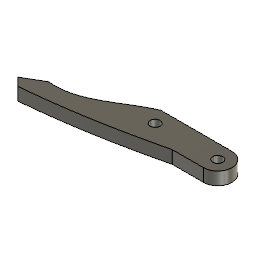
Gripper Holder 1.0 (Autodesk Fusion 360 design; units mm, degrees)
part number: 2026-08-19-22-23-44-975
Autodesk Fusion 360 part; units mm, degrees
sketch "Sketch1" plane through (0, 0, 0) normal (0, 0, 1) x (1, 0, 0)
  line L0 (-11, 0) -> (11, 0) construction
  circle A0 centre (-11, 0) radius 1.75
  circle A1 centre (-11, 0) radius 5
  circle A2 centre (11, 0) radius 1.75
  circle A3 centre (11, 0) radius 5
  line L1 (-11, 5) -> (11, 5)
  line L2 (11, -5) -> (-11, -5)
  dimension "d1" = 22
  dimension "d2" = 3.5
  dimension "d3" = 10
  dimension "d4" = 3.5
  dimension "d5" = 10
  constraint midpoint L0 origin
  constraint horizontal L0
  constraint coincident L0.start A0.centre
  constraint concentric A0 A1
  constraint coincident L0.end A2.centre
  constraint concentric A2 A3
  constraint coincident A1 L1.start
  constraint coincident A3 L1.end
  constraint tangent A3 L1
  constraint coincident A3 L2.start
  constraint coincident A1 L2.end
  constraint tangent A1 L2
  measures "d1" distance of L0.start L0.end
  measures "d2" diameter of A0
  measures "d3" diameter of A1
  measures "d4" diameter of A2
  measures "d5" diameter of A3
extrude "Extrude1" add sketch "Sketch1" along normal blind 4.5
sketch "Sketch2" plane through (0, 0, 4.5) normal (0, 0, 1) x (-1, 0, 0)
  circle A0 centre (-11, 0) radius 1.75
  circle A1 centre (11, 0) radius 1.75
  arc A2 (11, -5) -> (11, 5) centre (11, 0) ccw
  line L0 (11, 5) -> (-11, 5)
  arc A3 (-11, 5) -> (-11, -5) centre (-11, 0) ccw
  line L1 (-11, -5) -> (11, -5)
  line L2 (46.364, 12.87) -> (49.1808, 10.03)
  line L3 (49.1808, 10.03) -> (42.27, 6)
  line L4 (11, 0) -> (11, -5) construction
  spline S0 degree 5 poles (42.27, 6) (41.8597, 6.0483) (41.0377, 6.1242) (39.8004, 6.1754) (38.142, 6.1176) (36.0551, 5.832) (33.9568, 5.3324) (31.8528, 4.6259) (29.753, 3.7318) (27.6735, 2.6889) (25.6346, 1.5499) (23.6581, 0.3731) (21.7651, -0.7836) (19.9739, -1.8698) (18.2958, -2.85) (16.7347, -3.707) (15.5794, -4.2889) (14.7647, -4.667) (14.2444, -4.8933) (13.99, -5) knots 0 0 0 0 0 0 0.066667 0.133333 0.2 0.266667 0.333333 0.4 0.466667 0.533333 0.6 0.666667 0.733333 0.8 0.866667 0.933333 1 1 1 1 1 1
  line L5 (0, 0) -> (0, 5) construction
  spline S1 degree 5 poles (46.364, 12.87) (45.4848, 12.7904) (43.7223, 12.6243) (41.0656, 12.3544) (37.4975, 11.9526) (32.991, 11.3756) (28.4344, 10.7175) (23.8239, 9.9723) (19.158, 9.1377) (14.4396, 8.2182) (9.6729, 7.2207) (5.8243, 6.3656) (2.9193, 5.6943) (0.9744, 5.2336) (0, 5) knots 0 0 0 0 0 0 0.1 0.2 0.3 0.4 0.5 0.6 0.7 0.8 0.9 1 1 1 1 1 1
  line L6 (11, 0) -> (11, 5) construction
  line L7 (0, 5) -> (11, 5)
  line L8 (13.99, -5) -> (11, -5)
  point P0 (31.52, 4.45)
  point P1 (20.61, -1.48)
  point P2 (24.52, 10.07)
  dimension "d10" = 4
  dimension "d11" = 8
  dimension "d12" = 31.27
  dimension "d13" = 11
  dimension "d14" = 15.03
  dimension "d15" = 17.87
  dimension "d16" = 9.45
  dimension "d17" = 3.52
  dimension "d18" = 2.99
  dimension "d19" = 9.61
  dimension "d20" = 20.52
  dimension "d21" = 13.52
  dimension "d22" = 15.07
  constraint coincident A1.centre A2.centre
  constraint coincident A2.start L1.end
  constraint coincident L5.start origin
  constraint midpoint L0 L5.end
  constraint coincident A2.end L0.start
  constraint tangent A2 L8
  measures "d10" distance of L2.start L2.end
  measures "d11" distance of L2.end L3.end
  measures "d12" horizontal distance of L3.end A2.start
  measures "d13" vertical distance of L3.end A2.start
  measures "d14" vertical distance of L2.end A2.start
  measures "d15" vertical distance of L2.start A2.start
  measures "d16" vertical distance of A2.start P0
  measures "d17" vertical distance of A2.start P1
  measures "d18" distance of A2.start S0.end
  measures "d19" horizontal distance of A2.start P1
  measures "d20" horizontal distance of A2.start P0
  measures "d21" horizontal distance of P2 A2.end
  measures "d22" vertical distance of A3.end P2
extrude "Extrude2" add sketch "Sketch2" against normal up to surface (4.5 mm away) contours A2 L0 L2 L3 S0 S1 L7 L8
